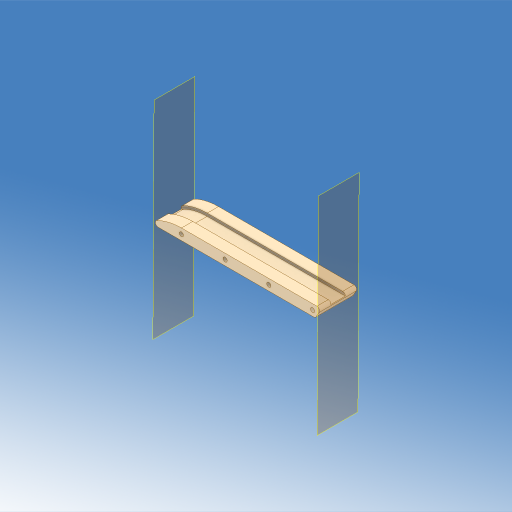
# Autodesk Inventor part: chain guide
Saved by Autodesk Inventor 2024 (Build 280153000, 153)
## iProperties
Created: 2023-03-01
Part Number: chain guide
Material: Polyethylene, High Density
Document SubType Name: Modeling
Designer: ralph
Density: 0.952 g/cm^3
Appearance: Smooth - Off-White
Author: ralph
Autodesk Inventor part; units mm, degrees
(part 1 of 2)
ref_plane "YZ Plane" through (0, 0, 0) normal (1, 0, 0) x (0, 1, 0)
ref_plane "XZ Plane" through (0, 0, 0) normal (0, 1, 0) x (-1, 0, 0)
ref_plane "XY Plane" through (0, 0, 0) normal (0, 0, 1) x (1, 0, 0)
ref_plane "Work Plane1" through (161.725, -21.8362, 0) normal (0, 0, 1) x (-0.4541702, 0.8909149, 0)
ref_plane "Work Plane2" through (-185.3421, -221.2521, 43.0784) normal (0, 0, -1) x (-0.1993348, 0.9799314, 0)
sketch "Sketch1" plane through (161.725, -21.8362, 0) normal (0, 0, 1) x (-0.4541702, 0.8909149, 0)
  circle A0 centre (-25.198, 87.6805) radius 3.175 projected
  line L0 (-137.9602, 56.9328) -> (35.8157, 235.3516) projected
  line L1 (82.5479, 91.7802) -> (42.7331, 68.5436) projected
  line L2 (134.3813, 156.1871) -> (107.8298, 115.7603) projected
  line L3 (-111.1407, 21.5887) -> (-101.5062, 29.8628) projected
  line L4 (-105.6433, 34.6801) -> (-115.2779, 26.406) projected
  line L5 (-3.5943, 192.0403) -> (-4.3034, 192.7309) projected
  line L6 (-3.5943, 192.0403) -> (-10.2226, 185.2349) projected
  line L7 (-10.9317, 185.9255) -> (-10.2226, 185.2349) projected
  arc A1 (2.942, 134.7748) -> (-78.867, 82.7393) centre (-35.4691, 104.837) ccw
  line L8 (2.942, 134.7748) -> (32.6751, 96.6265)
  arc A2 (44.4149, 71.1206) -> (32.6751, 96.6265) centre (-15.7529, 58.8814) ccw
  line L9 (44.4149, 71.1206) -> (83.6822, -121.9177)
  arc A3 (34.1459, -139.2082) -> (83.6822, -121.9177) centre (57.7385, -127.1951) ccw
  line L10 (34.1459, -139.2082) -> (-78.867, 82.7393)
  line L11 (86.7935, -121.2849) -> (47.5262, 71.7534)
  arc A4 (47.5262, 71.7534) -> (35.1793, 98.5783) centre (-15.7529, 58.8814) ccw
  line L12 (35.1793, 98.5783) -> (5.4462, 136.7266)
  arc A5 (5.4462, 136.7266) -> (-81.6964, 81.2986) centre (-35.4691, 104.837) ccw
  line L13 (-81.6964, 81.2986) -> (31.3166, -140.6489)
  arc A6 (31.3166, -140.6489) -> (86.7935, -121.2849) centre (57.7385, -127.1951) ccw
  line L14 (74.3484, -123.8164) -> (35.0811, 69.2219)
  arc A7 (35.0811, 69.2219) -> (25.1625, 90.7711) centre (-15.7529, 58.8814) ccw
  line L15 (25.1625, 90.7711) -> (-4.5706, 128.9194)
  arc A8 (-4.5706, 128.9194) -> (-70.379, 87.0612) centre (-35.4691, 104.837) ccw
  line L16 (-70.379, 87.0612) -> (42.6339, -134.8862)
  arc A9 (42.6339, -134.8862) -> (74.3484, -123.8164) centre (57.7385, -127.1951) ccw
  arc A10 (5.8406, 137.034) -> (-82.1419, 81.0717) centre (-35.4691, 104.837) ccw
  line L17 (5.8406, 137.034) -> (35.5737, 98.8857)
  arc A11 (48.0162, 71.8531) -> (35.5737, 98.8857) centre (-15.7529, 58.8814) ccw
  line L18 (48.0162, 71.8531) -> (87.2835, -121.1852)
  arc A12 (30.871, -140.8757) -> (87.2835, -121.1852) centre (57.7385, -127.1951) ccw
  line L19 (30.871, -140.8757) -> (-82.1419, 81.0717)
  line L20 (35.0811, 69.2219) -> (26.9658, 109.1164)
  circle A13 centre (57.7385, -127.1951) radius 44.45
  line L21 (76.5649, -86.9289) -> (65.8232, -81.9066)
  line L22 (5.092, 163.5049) -> (21.707, 97.431) projected
  line L23 (16.9598, 93.9553) -> (-30.1799, 123.0636) projected
  line L24 (-32.8692, 137.5188) -> (-4.5914, 166.5521) projected
  line L25 (29.8165, 96.4279) -> (15.4242, 153.6621) projected
  line L26 (20.7934, 156.6354) -> (60.85, 114.9227) projected
  line L27 (59.7201, 100.498) -> (42.2664, 90.3117) projected
  line L28 (16.7525, 188.4662) -> (29.5545, 201.6103) projected
  line L29 (102.7916, 142.7886) -> (91.8918, 126.1928) projected
  line L30 (66.3462, 120.2006) -> (40.7971, 146.806) projected
  line L31 (-106.6065, 61.8114) -> (-103.8347, 64.6572) projected
  line L32 (-88.1733, 62.7788) -> (-84.3051, 57.8167) projected
  line L33 (-71.9024, 23.6808) -> (-75.2673, 21.717) projected
  line L34 (-82.4286, 45.3973) -> (-80.2793, 47.2431) projected
  line L35 (-75.7066, 46.7865) -> (-69.9197, 39.3629) projected
  line L36 (41.0185, 151.4137) -> (46.0865, 155.7661) projected
  line L37 (41.1219, 161.5468) -> (35.4645, 156.6883) projected
  line L38 (31.1059, 156.8978) -> (17.9326, 170.6158) projected
  line L39 (-84.7406, 53.4561) -> (-87.3932, 51.1781) projected
  arc A14 (19.6429, 91.6626) -> (21.4459, 90.8569) centre (24.9298, 101.0743) ccw projected
  arc A15 (23.5785, 87.5163) -> (21.4459, 90.8569) centre (20.4213, 87.8518) ccw projected
  arc A16 (23.5785, 87.5163) -> (24.0318, 82.5663) centre (36.1917, 86.1757) ccw projected
  arc A17 (22.7005, 78.9892) -> (24.0318, 82.5663) centre (20.9881, 81.6628) ccw projected
  line L40 (22.7005, 78.9892) -> (6.0457, 68.3219) projected
  arc A18 (2.2151, 68.6304) -> (6.0457, 68.3219) centre (4.3333, 70.9955) ccw projected
  arc A19 (2.2151, 68.6304) -> (-6.0801, 71.8722) centre (-6.2676, 59.1587) ccw projected
  arc A20 (-8.9054, 73.6936) -> (-6.0801, 71.8722) centre (-6.0333, 75.0469) ccw projected
  line L41 (-8.9054, 73.6936) -> (-12.8049, 81.9696) projected
  arc A21 (-12.9858, 84.1944) -> (-12.8049, 81.9696) centre (-9.9328, 83.3229) ccw projected
  arc A22 (-12.9858, 84.1944) -> (-20.1115, 99.3174) centre (-25.198, 87.6805) ccw projected
  arc A23 (-21.712, 100.8733) -> (-20.1115, 99.3174) centre (-18.8398, 102.2266) ccw projected
  line L42 (-21.712, 100.8733) -> (-28.5783, 115.4459) projected
  arc A24 (-26.3647, 117.5067) -> (-28.5783, 115.4459) centre (-27.1422, 116.1226) ccw projected
  line L43 (-26.3647, 117.5067) -> (19.6429, 91.6626) projected
  line L44 (-65.6079, 77.0105) -> (-80.7722, 80.8743) projected
  line L45 (-82.4908, 86.5713) -> (-54.2131, 115.6046) projected
  line L46 (-42.2841, 112.6957) -> (-42.2475, 112.609) projected
  line L47 (-99.9792, 13.6685) -> (-98.0354, 10.338) projected
  line L48 (118.4433, 166.6195) -> (116.9435, 164.3359) projected
  line L49 (-124.3285, 43.6159) -> (-123.0701, 44.9079) projected
  line L50 (-120.8252, 44.9375) -> (-116.1944, 40.4272) projected
  line L51 (-43.1046, 108.967) -> (-65.0617, 90.1102) projected
  line L52 (-65.4017, 85.633) -> (-62.4154, 82.1557) projected
  ellipse E0 centre (81.3052, 191.0464) end of major axis (135.8081, 158.463) minor radius 63.4993 (134.3813, 156.1871) -> (35.8157, 235.3516) ccw projected
  ellipse E1 centre (44.1384, 157.5915) end of major axis (-21.2652, 196.6916) minor radius 76.1992 (82.5479, 91.7802) -> (107.8298, 115.7603) ccw projected
  ellipse E2 centre (-113.2093, 23.9973) end of major axis (-115.9344, 25.6265) minor radius 3.175 (-115.2779, 26.406) -> (-111.1407, 21.5887) ccw projected
  ellipse E3 centre (-103.5747, 32.2715) end of major axis (-106.2999, 33.9007) minor radius 3.175 (-101.5062, 29.8628) -> (-105.6433, 34.6801) ccw projected
  ellipse E4 centre (5.3104, 178.2592) end of major axis (-5.5902, 184.7759) minor radius 12.6999 (-0.7915, 167.1213) -> (2.6724, 165.8363) ccw projected
  ellipse E5 centre (2.0128, 162.7306) end of major axis (-0.7123, 164.3598) minor radius 3.175 (5.092, 163.5049) -> (2.6724, 165.8363) ccw projected
  ellipse E6 centre (18.6279, 96.6567) end of major axis (21.3531, 95.0276) minor radius 3.175 (16.9598, 93.9553) -> (21.707, 97.431) ccw projected
  ellipse E7 centre (-28.5118, 125.765) end of major axis (-25.7867, 124.1359) minor radius 3.175 (-31.6717, 126.0744) -> (-30.1799, 123.0636) ccw projected
  ellipse E8 centre (-44.3112, 127.3117) end of major axis (-55.2118, 133.8284) minor radius 12.6999 (-31.6717, 126.0744) -> (-33.338, 133.7052) ccw projected
  ellipse E9 centre (-30.5947, 135.3035) end of major axis (-27.8696, 133.6744) minor radius 3.175 (-32.8692, 137.5188) -> (-33.338, 133.7052) ccw projected
  ellipse E10 centre (-2.317, 164.3368) end of major axis (-5.0421, 165.966) minor radius 3.175 (-0.7915, 167.1213) -> (-4.5914, 166.5521) ccw projected
  ellipse E11 centre (32.8956, 97.2021) end of major axis (35.6207, 95.5729) minor radius 3.175 (29.8165, 96.4279) -> (32.2361, 94.0964) ccw projected
  ellipse E12 centre (18.5034, 154.4363) end of major axis (15.7782, 156.0655) minor radius 3.175 (20.7934, 156.6354) -> (15.4242, 153.6621) ccw projected
  ellipse E13 centre (58.56, 112.7236) end of major axis (55.8348, 114.3528) minor radius 3.175 (61.5424, 111.6347) -> (60.85, 114.9227) ccw projected
  ellipse E14 centre (73.4722, 107.2793) end of major axis (62.5716, 113.7959) minor radius 12.6999 (61.5424, 111.6347) -> (61.1902, 104.048) ccw projected
  ellipse E15 centre (58.1197, 103.2401) end of major axis (60.8449, 101.611) minor radius 3.175 (59.7201, 100.498) -> (61.1902, 104.048) ccw projected
  ellipse E16 centre (40.666, 93.0538) end of major axis (43.3911, 91.4247) minor radius 3.175 (38.4524, 90.7778) -> (42.2664, 90.3117) ccw projected
  ellipse E17 centre (20.2226, 172.8149) end of major axis (22.9478, 171.1857) minor radius 3.175 (17.2402, 173.9037) -> (17.9326, 170.6158) ccw projected
  ellipse E18 centre (5.3104, 178.2592) end of major axis (-5.5902, 184.7759) minor radius 12.6999 (17.2402, 173.9037) -> (16.2836, 184.6526) ccw projected
  ellipse E19 centre (19.0269, 186.251) end of major axis (21.7521, 184.6218) minor radius 3.175 (16.7525, 188.4662) -> (16.2836, 184.6526) ccw projected
  ellipse E20 centre (31.829, 199.395) end of major axis (29.1038, 201.0242) minor radius 3.175 (34.9594, 198.865) -> (29.5545, 201.6103) ccw projected
  ellipse E21 centre (81.29, 191.021) end of major axis (40.9578, 215.1327) minor radius 46.9895 (50.2522, 155.7412) -> (98.9449, 147.474) ccw projected
  ellipse E22 centre (100.1378, 144.5316) end of major axis (97.4127, 146.1608) minor radius 3.175 (102.7916, 142.7886) -> (98.9449, 147.474) ccw projected
  ellipse E23 centre (44.1233, 157.5662) end of major axis (-4.9294, 186.8912) minor radius 57.1494 (85.1993, 117.8311) -> (91.8918, 126.1928) ccw projected
  ellipse E24 centre (82.9173, 120.0386) end of major axis (85.6425, 118.4094) minor radius 3.175 (81.0283, 117.4867) -> (85.1993, 117.8311) ccw projected
  ellipse E25 centre (73.4722, 107.2793) end of major axis (62.5716, 113.7959) minor radius 12.6999 (81.0283, 117.4867) -> (69.6034, 119.3756) ccw projected
  ellipse E26 centre (68.6362, 122.3997) end of major axis (71.3614, 120.7705) minor radius 3.175 (66.3462, 120.2006) -> (69.6034, 119.3756) ccw projected
  ellipse E27 centre (-108.4072, 28.109) end of major axis (-132.9335, 42.7716) minor radius 28.5747 (-80.0217, 24.8241) -> (-83.1647, 41.5007) ccw projected
  ellipse E28 centre (-104.332, 59.5961) end of major axis (-101.6068, 57.967) minor radius 3.175 (-106.6065, 61.8114) -> (-104.7395, 56.4474) ccw projected
  ellipse E29 centre (-101.5603, 62.4419) end of major axis (-104.2854, 64.0711) minor radius 3.175 (-100.0348, 65.2264) -> (-103.8347, 64.6572) ccw projected
  ellipse E30 centre (-93.9329, 76.3643) end of major axis (-83.0323, 69.8476) minor radius 12.6999 (-100.0348, 65.2264) -> (-91.3284, 63.9343) ccw projected
  ellipse E31 centre (-90.6773, 60.8268) end of major axis (-93.4025, 62.456) minor radius 3.175 (-88.1733, 62.7788) -> (-91.3284, 63.9343) ccw projected
  ellipse E32 centre (-72.4237, 37.4109) end of major axis (-75.1489, 39.0401) minor radius 3.175 (-69.569, 36.0211) -> (-69.9197, 39.3629) ccw projected
  ellipse E33 centre (-58.1503, 30.4621) end of major axis (-69.0509, 36.9787) minor radius 12.6999 (-69.569, 36.0211) -> (-70.4323, 27.2308) ccw projected
  ellipse E34 centre (-73.5028, 26.4229) end of major axis (-70.7776, 24.7938) minor radius 3.175 (-71.9024, 23.6808) -> (-70.4323, 27.2308) ccw projected
  ellipse E35 centre (-76.8677, 24.4591) end of major axis (-74.1426, 22.8299) minor radius 3.175 (-80.0217, 24.8241) -> (-75.2673, 21.717) ccw projected
  ellipse E36 centre (-108.4072, 28.109) end of major axis (-132.9335, 42.7716) minor radius 28.5747 (-91.3563, 51.0389) -> (-104.7395, 56.4474) ccw projected
  ellipse E37 centre (81.29, 191.021) end of major axis (40.9578, 215.1327) minor radius 46.9895 (34.9594, 198.865) -> (41.7265, 165.6685) ccw projected
  ellipse E38 centre (-80.36, 42.9886) end of major axis (-83.0851, 44.6178) minor radius 3.175 (-82.4286, 45.3973) -> (-83.1647, 41.5007) ccw projected
  ellipse E39 centre (-78.2107, 44.8345) end of major axis (-80.9358, 46.4636) minor radius 3.175 (-75.7066, 46.7865) -> (-80.2793, 47.2431) ccw projected
  ellipse E40 centre (43.0871, 149.0051) end of major axis (45.8123, 147.3759) minor radius 3.175 (41.0185, 151.4137) -> (40.7971, 146.806) ccw projected
  ellipse E41 centre (48.155, 153.3574) end of major axis (45.4299, 154.9866) minor radius 3.175 (50.2522, 155.7412) -> (46.0865, 155.7661) ccw projected
  ellipse E42 centre (33.3959, 159.0969) end of major axis (36.1211, 157.4678) minor radius 3.175 (31.1059, 156.8978) -> (35.4645, 156.6883) ccw projected
  ellipse E43 centre (39.0533, 163.9555) end of major axis (36.3282, 165.5846) minor radius 3.175 (41.1219, 161.5468) -> (41.7265, 165.6685) ccw projected
  ellipse E44 centre (-86.8092, 55.8647) end of major axis (-89.5343, 57.4939) minor radius 3.175 (-84.7406, 53.4561) -> (-84.3051, 57.8167) ccw projected
  ellipse E45 centre (-89.4617, 53.5867) end of major axis (-86.7366, 51.9575) minor radius 3.175 (-91.3563, 51.0389) -> (-87.3932, 51.1781) ccw projected
  ellipse E46 centre (-79.9882, 83.951) end of major axis (-77.2631, 82.3218) minor radius 3.175 (-82.7772, 82.4337) -> (-80.7722, 80.8743) ccw projected
  ellipse E47 centre (-93.9329, 76.3643) end of major axis (-104.8335, 82.881) minor radius 12.6999 (-82.7772, 82.4337) -> (-82.9597, 82.7577) ccw projected
  ellipse E48 centre (-80.2164, 84.3561) end of major axis (-77.4912, 82.7269) minor radius 3.175 (-82.4908, 86.5713) -> (-82.9597, 82.7577) ccw projected
  ellipse E49 centre (-51.9386, 113.3893) end of major axis (-54.6638, 115.0185) minor radius 3.175 (-50.4131, 116.1738) -> (-54.2131, 115.6046) ccw projected
  ellipse E50 centre (-44.3112, 127.3117) end of major axis (-33.4106, 120.7951) minor radius 12.6999 (-50.4131, 116.1738) -> (-45.03, 114.6322) ccw projected
  ellipse E51 centre (-45.2097, 111.4623) end of major axis (-47.9349, 113.0915) minor radius 3.175 (-42.2841, 112.6957) -> (-45.03, 114.6322) ccw projected
  ellipse E52 centre (69.1742, 230.4776) end of major axis (66.4491, 232.1067) minor radius 3.175 (71.8221, 228.7255) -> (68.2422, 233.5127) ccw projected
  ellipse E53 centre (87.7091, 218.2134) end of major axis (71.3582, 227.9884) minor radius 19.0498 (71.8221, 228.7255) -> (69.7676, 224.6169) ccw projected
  ellipse E54 centre (66.7773, 225.6842) end of major axis (69.5025, 224.055) minor radius 3.175 (65.4394, 222.8049) -> (69.7676, 224.6169) ccw projected
  ellipse E55 centre (57.412, 205.529) end of major axis (41.0611, 215.3041) minor radius 19.0498 (65.4394, 222.8049) -> (61.0705, 224.2242) ccw projected
  ellipse E56 centre (61.6803, 227.3401) end of major axis (64.4054, 225.7109) minor radius 3.175 (60.1718, 230.1339) -> (61.0705, 224.2242) ccw projected
  ellipse E57 centre (81.29, 191.021) end of major axis (119.4421, 168.2127) minor radius 44.4495 (68.2422, 233.5127) -> (60.1718, 230.1339) ccw projected
  ellipse E58 centre (115.0715, 214.7362) end of major axis (117.7966, 213.107) minor radius 3.175 (114.2234, 211.6765) -> (117.6701, 216.5604) ccw projected
  ellipse E59 centre (109.1353, 193.3188) end of major axis (92.7844, 203.0938) minor radius 19.0498 (114.2234, 211.6765) -> (109.681, 212.3609) ccw projected
  ellipse E60 centre (109.772, 215.5345) end of major axis (112.4971, 213.9054) minor radius 3.175 (106.6201, 215.9172) -> (109.681, 212.3609) ccw projected
  ellipse E61 centre (87.7091, 218.2134) end of major axis (71.3582, 227.9884) minor radius 19.0498 (106.6201, 215.9172) -> (106.6199, 220.5109) ccw projected
  ellipse E62 centre (109.7718, 220.8938) end of major axis (107.0466, 222.5229) minor radius 3.175 (111.9627, 223.1917) -> (106.6199, 220.5109) ccw projected
  ellipse E63 centre (81.29, 191.021) end of major axis (119.4421, 168.2127) minor radius 44.4495 (117.6701, 216.5604) -> (111.9627, 223.1917) ccw projected
  ellipse E64 centre (-99.4065, 9.5378) end of major axis (-98.0439, 8.7232) minor radius 1.5875 (-98.7141, 8.1092) -> (-98.0354, 10.338) ccw projected
  ellipse E65 centre (-108.4072, 28.109) end of major axis (-127.4832, 39.5132) minor radius 22.2248 (-107.6415, 5.8974) -> (-98.7141, 8.1092) ccw projected
  ellipse E66 centre (-107.7509, 9.0705) end of major axis (-110.476, 10.6997) minor radius 3.175 (-108.8456, 12.0508) -> (-107.6415, 5.8974) ccw projected
  ellipse E67 centre (-113.2245, 23.972) end of major axis (-102.3239, 17.4553) minor radius 12.6999 (-108.8456, 12.0508) -> (-104.822, 14.4489) ccw projected
  ellipse E68 centre (-102.7214, 12.0682) end of major axis (-99.9962, 10.439) minor radius 3.175 (-99.9792, 13.6685) -> (-104.822, 14.4489) ccw projected
  ellipse E69 centre (114.2897, 166.0789) end of major axis (117.0148, 164.4497) minor radius 3.175 (111.1169, 165.9603) -> (116.9435, 164.3359) ccw projected
  ellipse E70 centre (92.0803, 165.2488) end of major axis (75.7294, 175.0238) minor radius 19.0498 (111.1169, 165.9603) -> (110.359, 170.6139) ccw projected
  ellipse E71 centre (113.4055, 171.5081) end of major axis (110.6804, 173.1372) minor radius 3.175 (112.7955, 174.6239) -> (110.359, 170.6139) ccw projected
  ellipse E72 centre (109.1353, 193.3188) end of major axis (92.7844, 203.0938) minor radius 19.0498 (112.7955, 174.6239) -> (117.1643, 176.0436) ccw projected
  ellipse E73 centre (118.5024, 173.1643) end of major axis (115.7773, 174.7935) minor radius 3.175 (121.3649, 171.7907) -> (117.1643, 176.0436) ccw projected
  ellipse E74 centre (81.29, 191.021) end of major axis (119.4421, 168.2127) minor radius 44.4495 (118.4433, 166.6195) -> (121.3649, 171.7907) ccw projected
  ellipse E75 centre (-121.9329, 43.8002) end of major axis (-123.2954, 44.6148) minor radius 1.5875 (-120.8252, 44.9375) -> (-123.0701, 44.9079) ccw projected
  ellipse E76 centre (-117.302, 39.29) end of major axis (-118.6646, 40.1046) minor radius 1.5875 (-116.3137, 38.0477) -> (-116.1944, 40.4272) ccw projected
  ellipse E77 centre (-108.4072, 28.109) end of major axis (-119.3078, 34.6257) minor radius 12.6999 (-116.3137, 38.0477) -> (-118.8274, 35.3692) ccw projected
  ellipse E78 centre (-113.2245, 23.972) end of major axis (-102.3239, 17.4553) minor radius 12.6999 (-118.8274, 35.3692) -> (-124.3475, 30.1012) ccw projected
  ellipse E79 centre (-127.1283, 31.6335) end of major axis (-129.8534, 33.2627) minor radius 3.175 (-130.2485, 32.2209) -> (-124.3475, 30.1012) ccw projected
  ellipse E80 centre (-108.4072, 28.109) end of major axis (-127.4832, 39.5132) minor radius 22.2248 (-124.3285, 43.6159) -> (-130.2485, 32.2209) ccw projected
  ellipse E81 centre (29.598, 81.6735) end of major axis (18.6974, 88.1902) minor radius 12.6999 (38.4524, 90.7778) -> (32.2361, 94.0964) ccw projected
  ellipse E82 centre (-62.9931, 87.7016) end of major axis (-60.2679, 86.0724) minor radius 3.175 (-65.0617, 90.1102) -> (-65.4017, 85.633) ccw projected
  ellipse E83 centre (-64.824, 80.0872) end of major axis (-62.0989, 78.458) minor radius 3.175 (-65.6079, 77.0105) -> (-62.4154, 82.1557) ccw projected
  ellipse E84 centre (-48.9751, 61.6327) end of major axis (-51.7002, 63.2618) minor radius 3.175 (-46.5664, 63.7012) -> (-48.1912, 64.7093) ccw projected
  line L53 (-46.5664, 63.7012) -> (-45.0469, 61.9319) projected
  ellipse E85 centre (-42.6383, 64.0005) end of major axis (-39.9132, 62.3713) minor radius 3.175 (-45.0469, 61.9319) -> (-40.6714, 61.5081) ccw projected
  ellipse E86 centre (-38.7045, 59.0157) end of major axis (-35.9794, 57.3866) minor radius 3.175 (-37.9206, 62.0924) -> (-40.6714, 61.5081) ccw projected
  line L54 (-37.9206, 62.0924) -> (-29.3488, 59.9083) projected
  line L55 (-78.8602, 72.5238) -> (-48.1912, 64.7093) projected
  ellipse E87 centre (2.465, 188.3722) end of major axis (0.5563, 189.5157) minor radius 2.225 projected
  ellipse E88 centre (-6.396, 179.2744) end of major axis (-4.4874, 178.1309) minor radius 2.225 projected
  ellipse E89 centre (-6.396, 179.2744) end of major axis (-11.4572, 182.3067) minor radius 5.8999 (-10.8256, 183.1717) -> (-0.6248, 178.0483) ccw projected
  ellipse E90 centre (5.2441, 176.8013) end of major axis (10.3911, 173.7176) minor radius 5.9999 (3.8429, 182.6354) -> (-0.6248, 178.0483) ccw projected
  ellipse E91 centre (2.465, 188.3722) end of major axis (-2.5962, 191.4045) minor radius 5.8999 (3.8429, 182.6354) -> (-1.5477, 192.6974) ccw projected
  ellipse E92 centre (-2.908, 194.1636) end of major axis (-4.6236, 195.1915) minor radius 2 (-4.3034, 192.7309) -> (-1.5477, 192.6974) ccw projected
  ellipse E93 centre (-12.3272, 184.4928) end of major axis (-10.6115, 183.4649) minor radius 2 (-10.8256, 183.1717) -> (-10.9317, 185.9255) ccw projected
  ellipse E94 centre (-108.392, 28.1344) end of major axis (-72.9651, 6.9552) minor radius 41.2746 (-137.9602, 56.9328) -> (-87.5869, -7.5134) ccw projected
  arc A25 (42.7331, 68.5436) -> (42.2932, 68.2869) centre (41.3036, 70.4877) ccw projected
  circle A26 centre (-43.1479, 88.299) radius 12.7 projected
  ellipse E95 centre (-45.1732, 111.3756) end of major axis (-47.8983, 113.0048) minor radius 3.175 (-43.1046, 108.967) -> (-42.2475, 112.609) ccw projected
  ellipse E96 centre (-30.1327, 56.8316) end of major axis (-32.8579, 58.4608) minor radius 3.175 (-26.9614, 56.6789) -> (-29.3488, 59.9083) ccw projected
  line L56 (42.2932, 68.2869) -> (-87.5869, -7.5134) projected
  ellipse E97 centre (-14.2761, 56.0678) end of major axis (-25.1767, 62.5845) minor radius 12.6999 (-26.9614, 56.6789) -> (-26.5581, 52.8365) ccw projected
  ellipse E98 centre (-29.6286, 52.0287) end of major axis (-26.9035, 50.3995) minor radius 3.175 (-28.0282, 49.2865) -> (-26.5581, 52.8365) ccw projected
  line L57 (-28.0282, 49.2865) -> (-45.482, 39.1002) projected
  ellipse E99 centre (-47.0824, 41.8423) end of major axis (-44.3572, 40.2132) minor radius 3.175 (-49.296, 39.5663) -> (-45.482, 39.1002) ccw projected
  ellipse E100 centre (-58.1503, 30.4621) end of major axis (-69.0509, 36.9787) minor radius 12.6999 (-49.296, 39.5663) -> (-60.7548, 42.8921) ccw projected
  ellipse E101 centre (-61.4059, 45.9996) end of major axis (-58.6808, 44.3704) minor radius 3.175 (-63.9099, 44.0476) -> (-60.7548, 42.8921) ccw projected
  line L58 (-63.9099, 44.0476) -> (-82.1636, 67.4635) projected
  ellipse E102 centre (-79.6595, 69.4155) end of major axis (-76.9344, 67.7863) minor radius 3.175 (-82.5142, 70.8052) -> (-82.1636, 67.4635) ccw projected
  ellipse E103 centre (-93.9329, 76.3643) end of major axis (-83.0323, 69.8476) minor radius 12.6999 (-82.5142, 70.8052) -> (-82.5019, 70.8306) ccw projected
  ellipse E104 centre (-79.6441, 69.4471) end of major axis (-76.919, 67.818) minor radius 3.175 (-78.8602, 72.5238) -> (-82.5019, 70.8306) ccw projected
  point P0 (92.9048, 134.1658)
  point P1 (66.1574, -83.5497)
  point P2 (80.1923, -88.8333)
  point P3 (-35.4703, 104.8623)
  point P4 (57.7373, -127.1698)
  dimension "d3" = 88.9
  dimension "d0" = 3.175
  dimension "d2" = 12.7
  constraints: 28 end point, 24 point on circle, 12 centre point, 3 point on line, 1 coincident, 1 collinear, 131 other
  measures "d0" distance between parallel lines of L9 L11
  measures "d2" distance between parallel lines of L11 L14
extrude "Extrusion1" add sketch "Sketch1" along normal up to surface (43.0784 mm away) contours A13 L9 L1 L11 | L56 A25 L1 L9 L21 L14 | L14 L20 L25 E11 E81 A2 L9 L1 A25 L56 | L14 L21 A13 | L1 L9 A2 E81 E16 A4 L11 | L20 L12 A4 E16 E81 A2 L8 | L8 A2 E81 E11 L25 L20
fillet "Fillet1" radius 3.175 1 edges at (52.2645, -47.3693, 21.5392)
ref_plane "Work Plane3" through (204.4469, 89.9538, 21.5392) normal (0, 0, 1) x (-0.622646, 0.7825036, 0)
sketch "Sketch3" plane through (204.4469, 89.9538, 21.5392) normal (0, 0, 1) x (-0.622646, 0.7825036, 0)
  line L0 (-184.7381, 186.3043) -> (21.1154, 326.503) projected
  line L1 (38.291, 176.4975) -> (-148.2221, 113.1103) projected
  line L2 (101.9227, 229.2796) -> (67.8456, 194.9568) projected
  line L3 (-168.5961, 151.8687) -> (-157.5055, 158.0564) projected
  line L4 (-154.4116, 152.5111) -> (-165.5022, 146.3234) projected
  line L5 (-121.6496, 199.8402) -> (-55.1465, -40.1805)
  arc A0 (-55.1465, -40.1805) -> (-3.1929, -33.1162) centre (-29.65, -33.1162) ccw
  line L6 (-3.1929, -33.1162) -> (-3.1929, 163.8755)
  arc A1 (-3.1929, 163.8755) -> (-9.611, 191.2017) centre (-64.575, 163.8755) ccw
  line L7 (-9.611, 191.2017) -> (-31.1431, 234.5113)
  arc A2 (-31.1431, 234.5113) -> (-121.6496, 199.8402) centre (-74.735, 212.8389) ccw
  line L8 (-125.1888, 198.8596) -> (-58.6857, -41.1611)
  arc A3 (-58.6857, -41.1611) -> (0.4796, -33.1162) centre (-29.65, -33.1162) ccw
  line L9 (0.4796, -33.1162) -> (0.4796, 163.8755)
  arc A4 (0.4796, 163.8755) -> (-6.3225, 192.8367) centre (-64.575, 163.8755) ccw
  line L10 (-6.3225, 192.8367) -> (-27.8546, 236.1463)
  arc A5 (-27.8546, 236.1463) -> (-125.1888, 198.8596) centre (-74.735, 212.8389) ccw
  line L11 (0, 0) -> (0, 163.8755) projected
  arc A6 (0, 0) -> (-12.7, 7.9752) centre (-29.65, -33.1162) ccw projected
  arc A7 (0, 163.8755) -> (-6.6784, 192.4746) centre (-64.575, 163.8755) ccw projected
  arc A8 (-6.6784, 192.4746) -> (-12.7, 191.0684) centre (-9.525, 191.0684) ccw projected
  line L12 (-12.7, 191.0684) -> (-12.7, 7.9752) projected
  line L13 (0, 0) -> (-3.1929, 2.2689)
  line L14 (-3.1929, 2.6025) -> (-3.1929, 163.8755)
  line L15 (-65.6726, 244.3466) -> (-32.1751, 267.1605) projected
  line L16 (-126.6144, 140.5738) -> (-130.3033, 139.3202) projected
  line L17 (-153.0212, 184.857) -> (-149.7379, 187.0931) projected
  line L18 (68.3161, 222.4688) -> (54.3269, 208.3787) projected
  line L19 (17.679, 189.6125) -> (-1.455, 183.1097) projected
  line L20 (-30.4188, 173.2663) -> (-49.5528, 166.7635) projected
  line L21 (-123.6965, 189.8236) -> (-95.2006, 176.0525) projected
  line L22 (-78.5166, 156.9201) -> (-97.6506, 150.4173) projected
  line L23 (-114.7225, 158.9387) -> (-127.9422, 185.5233) projected
  line L24 (-65.5928, 218.8876) -> (-28.5919, 184.15) projected
  line L25 (-62.7617, 175.5508) -> (-64.1496, 182.4577) projected
  line L26 (-69.3588, 208.3833) -> (-70.8787, 215.9475) projected
  line L27 (-79.8467, 221.8984) -> (-79.8282, 221.8061) projected
  line L28 (-109.8158, 191.5786) -> (-123.9055, 198.3877) projected
  line L29 (-124.4541, 204.3129) -> (-90.9565, 227.1268) projected
  line L30 (-134.7651, 182.1305) -> (-131.9637, 176.497) projected
  line L31 (28.0995, 207.5989) -> (8.3665, 238.7632) projected
  line L32 (-12.4358, 191.5849) -> (-15.1305, 250.5393) projected
  line L33 (-9.2763, 252.3828) -> (21.6616, 203.5225) projected
  line L34 (-23.2934, 262.2442) -> (-20.1826, 194.1844) projected
  line L35 (-25.5274, 191.7247) -> (-65.9188, 229.6454) projected
  line L36 (-133.2597, 172.3107) -> (-136.3131, 170.6071) projected
  line L37 (0.8815, 250.5843) -> (-9.293, 266.6528) projected
  line L38 (11.6232, 253.1434) -> (5.1109, 249.5101) projected
  line L39 (-132.6005, 163.9528) -> (-130.1263, 165.3331) projected
  line L40 (-125.7365, 163.9741) -> (-121.5455, 155.546) projected
  line L41 (9.502, 243.2343) -> (15.3358, 246.4891) projected
  line L42 (-174.0146, 170.5592) -> (-172.5239, 171.5744) projected
  line L43 (-170.3182, 171.156) -> (-166.6794, 165.8131) projected
  line L44 (-156.1236, 136.3592) -> (-154.8827, 132.708) projected
  line L45 (88.404, 242.7015) -> (86.4791, 240.7627) projected
  line L46 (-81.394, 218.4081) -> (-106.6692, 204.3065) projected
  line L47 (-107.8949, 199.987) -> (-105.6617, 195.9842) projected
  line L48 (-85.6578, 171.4408) -> (-77.6934, 167.5919) projected
  line L49 (-93.8094, 174.7408) -> (-92.6731, 172.7041) projected
  line L50 (-59.8451, 191.0194) -> (-69.0187, 207.4618) projected
  line L51 (-62.5837, 185.8558) -> (-61.0708, 186.6999) projected
  ellipse E0 centre (0.0819, 301.4333) end of major axis (-4.2511, 305.4378) minor radius 5.8999 (0.2886, 295.537) -> (-2.9881, 306.4717) ccw projected
  ellipse E1 centre (0.0779, 301.429) end of major axis (1.7119, 299.9189) minor radius 2.225 projected
  ellipse E2 centre (-161.5039, 152.1899) end of major axis (-131.0096, 124.3739) minor radius 41.2746 (-184.7381, 186.3043) -> (-148.2221, 113.1103) ccw projected
  ellipse E3 centre (13.7708, 248.6444) end of major axis (-42.5262, 299.997) minor radius 76.1992 (38.291, 176.4975) -> (67.8456, 194.9568) ccw projected
  ellipse E4 centre (56.8604, 274.0192) end of major axis (103.7746, 231.2254) minor radius 63.4993 (101.9227, 229.2796) -> (21.1154, 326.503) ccw projected
  ellipse E5 centre (-155.9586, 155.2837) end of major axis (-158.3043, 157.4234) minor radius 3.175 (-154.4116, 152.5111) -> (-157.5055, 158.0564) ccw projected
  ellipse E6 centre (-167.0491, 149.0961) end of major axis (-169.3948, 151.2358) minor radius 3.175 (-168.5961, 151.8687) -> (-165.5022, 146.3234) ccw projected
  ellipse E7 centre (-137.7011, 196.5915) end of major axis (-147.0839, 205.1503) minor radius 12.6999 (-145.9007, 186.8934) -> (-137.6266, 183.8918) ccw projected
  ellipse E8 centre (-111.7866, 144.4778) end of major axis (-102.4037, 135.919) minor radius 12.6999 (-101.2951, 151.6343) -> (-111.861, 157.1775) ccw projected
  ellipse E9 centre (-127.6361, 143.58) end of major axis (-125.2904, 141.4403) minor radius 3.175 (-126.6144, 140.5738) -> (-124.4662, 143.7595) ccw projected
  ellipse E10 centre (-131.3249, 142.3263) end of major axis (-128.9792, 140.1866) minor radius 3.175 (-134.3428, 143.3127) -> (-130.3033, 139.3202) ccw projected
  ellipse E11 centre (-151.234, 182.2328) end of major axis (-148.8883, 180.0931) minor radius 3.175 (-153.0212, 184.857) -> (-152.261, 179.2285) ccw projected
  ellipse E12 centre (-147.9506, 184.4689) end of major axis (-150.2963, 186.6086) minor radius 3.175 (-145.9007, 186.8934) -> (-149.7379, 187.0931) ccw projected
  ellipse E13 centre (-78.9197, 236.6252) end of major axis (-69.5369, 228.0664) minor radius 12.6999 (-66.7804, 232.8932) -> (-66.8923, 240.703) ccw projected
  ellipse E14 centre (-63.8854, 241.7224) end of major axis (-61.5397, 239.5827) minor radius 3.175 (-65.6726, 244.3466) -> (-66.8923, 240.703) ccw projected
  ellipse E15 centre (-30.3878, 264.5363) end of major axis (-32.7335, 266.676) minor radius 3.175 (-28.3379, 266.9608) -> (-32.1751, 267.1605) ccw projected
  ellipse E16 centre (-20.1383, 276.6589) end of major axis (-10.7554, 268.1001) minor radius 12.6999 (-28.3379, 266.9608) -> (-25.1997, 265.0112) ccw projected
  ellipse E17 centre (56.8604, 274.0192) end of major axis (91.5769, 242.3518) minor radius 46.9895 (19.413, 245.6343) -> (65.4806, 227.8269) ccw projected
  ellipse E18 centre (66.063, 224.7058) end of major axis (63.7173, 226.8455) minor radius 3.175 (68.3161, 222.4688) -> (65.4806, 227.8269) ccw projected
  ellipse E19 centre (13.7708, 248.6444) end of major axis (-28.4519, 287.1588) minor radius 57.1494 (46.1019, 201.5188) -> (54.3269, 208.3787) ccw projected
  ellipse E20 centre (44.3058, 204.1369) end of major axis (46.6515, 201.9972) minor radius 3.175 (41.946, 202.0128) -> (46.1019, 201.5188) ccw projected
  ellipse E21 centre (32.5068, 193.5164) end of major axis (41.8897, 184.9576) minor radius 12.6999 (21.6847, 200.1625) -> (19.8272, 192.7982) ccw projected
  ellipse E22 centre (16.6573, 192.6186) end of major axis (19.003, 190.4789) minor radius 3.175 (17.679, 189.6125) -> (19.8272, 192.7982) ccw projected
  ellipse E23 centre (-2.4766, 186.1159) end of major axis (-0.1309, 183.9762) minor radius 3.175 (-5.0995, 184.3267) -> (-1.455, 183.1097) ccw projected
  ellipse E24 centre (-15.591, 177.1702) end of major axis (-6.2081, 168.6114) minor radius 12.6999 (-5.0995, 184.3267) -> (-10.5295, 188.8179) ccw projected
  ellipse E25 centre (-31.4405, 176.2724) end of major axis (-29.0948, 174.1327) minor radius 3.175 (-30.4188, 173.2663) -> (-28.2706, 176.452) ccw projected
  ellipse E26 centre (-50.5744, 169.7696) end of major axis (-48.2287, 167.63) minor radius 3.175 (-53.1973, 167.9805) -> (-49.5528, 166.7635) ccw projected
  ellipse E27 centre (-79.0749, 164.7332) end of major axis (-81.4206, 166.8729) minor radius 3.175 (-75.9976, 163.9514) -> (-77.6934, 167.5919) ccw projected
  ellipse E28 centre (-63.6888, 160.824) end of major axis (-54.3059, 152.2652) minor radius 12.6999 (-75.9976, 163.9514) -> (-76.3684, 160.1057) ccw projected
  ellipse E29 centre (-79.5383, 159.9262) end of major axis (-77.1926, 157.7865) minor radius 3.175 (-78.5166, 156.9201) -> (-76.3684, 160.1057) ccw projected
  ellipse E30 centre (-98.6722, 153.4234) end of major axis (-96.3265, 151.2837) minor radius 3.175 (-101.2951, 151.6343) -> (-97.6506, 150.4173) ccw projected
  ellipse E31 centre (-111.8796, 160.3524) end of major axis (-109.5339, 158.2127) minor radius 3.175 (-114.7225, 158.9387) -> (-111.861, 157.1775) ccw projected
  ellipse E32 centre (-63.6888, 160.824) end of major axis (-54.3059, 152.2652) minor radius 12.6999 (-53.1973, 167.9805) -> (-60.4569, 173.1058) ccw projected
  ellipse E33 centre (-59.649, 176.1762) end of major axis (-57.3033, 174.0365) minor radius 3.175 (-62.7617, 175.5508) -> (-60.4569, 173.1058) ccw projected
  ellipse E34 centre (-67.766, 216.5729) end of major axis (-70.1117, 218.7126) minor radius 3.175 (-65.5928, 218.8876) -> (-70.8787, 215.9475) ccw projected
  ellipse E35 centre (-122.524, 201.2463) end of major axis (-120.1783, 199.1066) minor radius 3.175 (-125.5594, 200.3154) -> (-123.9055, 198.3877) ccw projected
  ellipse E36 centre (-137.7011, 196.5915) end of major axis (-128.3183, 188.0328) minor radius 12.6999 (-125.5594, 200.3154) -> (-125.6737, 200.6693) ccw projected
  ellipse E37 centre (-122.6668, 201.6887) end of major axis (-120.3211, 199.549) minor radius 3.175 (-124.4541, 204.3129) -> (-125.6737, 200.6693) ccw projected
  ellipse E38 centre (-89.1692, 224.5026) end of major axis (-91.5149, 226.6423) minor radius 3.175 (-87.1193, 226.9271) -> (-90.9565, 227.1268) ccw projected
  ellipse E39 centre (-78.9197, 236.6252) end of major axis (-88.3025, 245.184) minor radius 12.6999 (-87.1193, 226.9271) -> (-82.1515, 224.3434) ccw projected
  ellipse E40 centre (-82.9595, 221.273) end of major axis (-85.3052, 223.4127) minor radius 3.175 (-79.8467, 221.8984) -> (-82.1515, 224.3434) ccw projected
  ellipse E41 centre (-111.7866, 144.4778) end of major axis (-102.4037, 135.919) minor radius 12.6999 (-121.868, 152.2014) -> (-124.4662, 143.7595) ccw projected
  ellipse E42 centre (-137.608, 180.7169) end of major axis (-139.9537, 182.8566) minor radius 3.175 (-134.7651, 182.1305) -> (-137.6266, 183.8918) ccw projected
  ellipse E43 centre (-124.3883, 154.1323) end of major axis (-126.7341, 156.272) minor radius 3.175 (-121.868, 152.2014) -> (-121.5455, 155.546) ccw projected
  ellipse E44 centre (-6.6105, 268.3513) end of major axis (-4.2648, 266.2116) minor radius 3.175 (-9.3161, 270.0128) -> (-9.293, 266.6528) ccw projected
  ellipse E45 centre (30.7819, 209.2973) end of major axis (33.1276, 207.1577) minor radius 3.175 (28.0995, 207.5989) -> (31.1269, 206.1412) ccw projected
  ellipse E46 centre (-9.2642, 191.7298) end of major axis (-6.9185, 189.5901) minor radius 3.175 (-12.4358, 191.5849) -> (-10.5295, 188.8179) ccw projected
  ellipse E47 centre (-11.9588, 250.6843) end of major axis (-14.3045, 252.824) minor radius 3.175 (-9.2763, 252.3828) -> (-15.1305, 250.5393) ccw projected
  ellipse E48 centre (18.9791, 201.824) end of major axis (16.6334, 203.9637) minor radius 3.175 (21.6847, 200.1625) -> (21.6616, 203.5225) ccw projected
  ellipse E49 centre (-26.4651, 262.0993) end of major axis (-28.8108, 264.239) minor radius 3.175 (-23.2934, 262.2442) -> (-25.1997, 265.0112) ccw projected
  ellipse E50 centre (-23.3543, 194.0394) end of major axis (-21.0085, 191.8998) minor radius 3.175 (-25.5274, 191.7247) -> (-20.1826, 194.1844) ccw projected
  ellipse E51 centre (-63.7456, 231.9601) end of major axis (-61.3999, 229.8205) minor radius 3.175 (-66.7804, 232.8932) -> (-65.9188, 229.6454) ccw projected
  ellipse E52 centre (-161.5039, 152.1899) end of major axis (-140.3925, 132.9327) minor radius 28.5747 (-134.3428, 143.3127) -> (-134.0986, 160.2811) ccw projected
  ellipse E53 centre (-161.5039, 152.1899) end of major axis (-140.3925, 132.9327) minor radius 28.5747 (-140.2244, 171.2608) -> (-152.261, 179.2285) ccw projected
  ellipse E54 centre (56.8604, 274.0192) end of major axis (91.5769, 242.3518) minor radius 46.9895 (13.0232, 290.9411) -> (13.0373, 257.0618) ccw projected
  ellipse E55 centre (-134.8066, 175.0833) end of major axis (-137.1523, 177.223) minor radius 3.175 (-133.2597, 172.3107) -> (-131.9637, 176.497) ccw projected
  ellipse E56 centre (-137.86, 173.3798) end of major axis (-135.5143, 171.2401) minor radius 3.175 (-140.2244, 171.2608) -> (-136.3131, 170.6071) ccw projected
  ellipse E57 centre (10.0762, 255.9161) end of major axis (7.7305, 258.0558) minor radius 3.175 (11.6232, 253.1434) -> (13.0373, 257.0618) ccw projected
  ellipse E58 centre (3.5639, 252.2827) end of major axis (5.9096, 250.1431) minor radius 3.175 (0.8815, 250.5843) -> (5.1109, 249.5101) ccw projected
  ellipse E59 centre (-30.765, 181.8352) end of major axis (-33.1107, 183.9749) minor radius 3.175 (-27.7302, 180.9022) -> (-28.5919, 184.15) ccw projected
  ellipse E60 centre (-128.5794, 162.5605) end of major axis (-130.9251, 164.7002) minor radius 3.175 (-125.7365, 163.9741) -> (-130.1263, 165.3331) ccw projected
  ellipse E61 centre (-131.0535, 161.1801) end of major axis (-133.3992, 163.3198) minor radius 3.175 (-132.6005, 163.9528) -> (-134.0986, 160.2811) ccw projected
  ellipse E62 centre (16.8827, 243.7164) end of major axis (14.537, 245.8561) minor radius 3.175 (19.413, 245.6343) -> (15.3358, 246.4891) ccw projected
  ellipse E63 centre (11.049, 240.4616) end of major axis (13.3947, 238.3219) minor radius 3.175 (9.502, 243.2343) -> (8.3665, 238.7632) ccw projected
  ellipse E64 centre (-161.5039, 152.1899) end of major axis (-177.9238, 167.1677) minor radius 22.2248 (-174.0146, 170.5592) -> (-182.0872, 160.573) ccw projected
  ellipse E65 centre (-171.6303, 170.2624) end of major axis (-172.8032, 171.3322) minor radius 1.5875 (-170.3182, 171.156) -> (-172.5239, 171.5744) ccw projected
  ellipse E66 centre (-167.9915, 164.9195) end of major axis (-169.1643, 165.9894) minor radius 1.5875 (-167.2706, 163.5051) -> (-166.6794, 165.8131) ccw projected
  ellipse E67 centre (-161.5039, 152.1899) end of major axis (-152.121, 143.6311) minor radius 12.6999 (-167.2706, 163.5051) -> (-170.2677, 161.3814) ccw projected
  ellipse E68 centre (-167.0491, 149.0961) end of major axis (-176.432, 157.6549) minor radius 12.6999 (-170.2677, 161.3814) -> (-176.7272, 157.3196) ccw projected
  ellipse E69 centre (-179.1467, 159.3754) end of major axis (-181.4924, 161.5151) minor radius 3.175 (-182.0872, 160.573) -> (-176.7272, 157.3196) ccw projected
  ellipse E70 centre (-159.1297, 135.3376) end of major axis (-156.784, 133.1979) minor radius 3.175 (-156.1236, 136.3592) -> (-160.7136, 138.0893) ccw projected
  ellipse E71 centre (-156.3857, 132.1972) end of major axis (-155.2129, 131.1274) minor radius 1.5875 (-155.992, 130.6593) -> (-154.8827, 132.708) ccw projected
  ellipse E72 centre (-161.5039, 152.1899) end of major axis (-177.9238, 167.1677) minor radius 22.2248 (-165.1811, 130.2714) -> (-155.992, 130.6593) ccw projected
  ellipse E73 centre (-164.6558, 133.4026) end of major axis (-167.0015, 135.5423) minor radius 3.175 (-165.1345, 136.5413) -> (-165.1811, 130.2714) ccw projected
  ellipse E74 centre (-167.0491, 149.0961) end of major axis (-176.432, 157.6549) minor radius 12.6999 (-165.1345, 136.5413) -> (-160.7136, 138.0893) ccw projected
  ellipse E75 centre (68.571, 299.3863) end of major axis (82.6453, 286.5482) minor radius 19.0498 (55.0983, 312.8544) -> (52.2661, 309.2377) ccw projected
  ellipse E76 centre (49.5486, 310.8796) end of major axis (51.8943, 308.7399) minor radius 3.175 (47.6635, 308.3248) -> (52.2661, 309.2377) ccw projected
  ellipse E77 centre (36.3535, 292.9958) end of major axis (50.4278, 280.1577) minor radius 19.0498 (47.6635, 308.3248) -> (43.6653, 310.5865) ccw projected
  ellipse E78 centre (44.8839, 313.5183) end of major axis (47.2296, 311.3786) minor radius 3.175 (43.9626, 316.5567) -> (43.6653, 310.5865) ccw projected
  ellipse E79 centre (56.8604, 274.0192) end of major axis (89.7003, 244.0636) minor radius 44.4495 (52.5445, 318.259) -> (43.9626, 316.5567) ccw projected
  ellipse E80 centre (52.8528, 315.099) end of major axis (50.5071, 317.2387) minor radius 3.175 (55.0983, 312.8544) -> (52.5445, 318.259) ccw projected
  ellipse E81 centre (84.6049, 270.7204) end of major axis (98.6791, 257.8822) minor radius 19.0498 (93.2503, 287.6954) -> (88.9354, 289.2715) ccw projected
  ellipse E82 centre (89.6572, 292.3633) end of major axis (92.0029, 290.2236) minor radius 3.175 (86.6449, 293.3666) -> (88.9354, 289.2715) ccw projected
  ellipse E83 centre (68.571, 299.3863) end of major axis (82.6453, 286.5482) minor radius 19.0498 (86.6449, 293.3666) -> (87.5604, 297.8681) ccw projected
  ellipse E84 centre (90.7252, 297.6151) end of major axis (88.3795, 299.7548) minor radius 3.175 (93.3302, 299.4301) -> (87.5604, 297.8681) ccw projected
  ellipse E85 centre (56.8604, 274.0192) end of major axis (89.7003, 244.0636) minor radius 44.4495 (97.6012, 291.7943) -> (93.3302, 299.4301) ccw projected
  ellipse E86 centre (94.6912, 290.5246) end of major axis (97.0369, 288.3849) minor radius 3.175 (93.2503, 287.6954) -> (97.6012, 291.7943) ccw projected
  ellipse E87 centre (56.8604, 274.0192) end of major axis (89.7003, 244.0636) minor radius 44.4495 (88.404, 242.7015) -> (92.2978, 247.1865) ccw projected
  ellipse E88 centre (84.226, 242.9997) end of major axis (86.5717, 240.86) minor radius 3.175 (81.0932, 243.5159) -> (86.4791, 240.7627) ccw projected
  ellipse E89 centre (62.2968, 246.6133) end of major axis (76.3711, 233.7752) minor radius 19.0498 (81.0932, 243.5159) -> (81.2782, 248.2272) ccw projected
  ellipse E90 centre (84.4418, 248.4961) end of major axis (82.0961, 250.6358) minor radius 3.175 (84.4651, 251.671) -> (81.2782, 248.2272) ccw projected
  ellipse E91 centre (84.6049, 270.7204) end of major axis (98.6791, 257.8822) minor radius 19.0498 (84.4651, 251.671) -> (89.0292, 252.1913) ccw projected
  ellipse E92 centre (89.7666, 249.1032) end of major axis (87.4208, 251.2429) minor radius 3.175 (92.2978, 247.1865) -> (89.0292, 252.1913) ccw projected
  ellipse E93 centre (-86.3214, 186.8641) end of major axis (-85.3831, 186.0082) minor radius 1.27 projected
  ellipse E94 centre (-75.2309, 193.0517) end of major axis (-74.2926, 192.1958) minor radius 1.27 projected
  ellipse E95 centre (-92.5092, 197.9547) end of major axis (-91.5709, 197.0988) minor radius 1.27 projected
  ellipse E96 centre (-81.4186, 204.1423) end of major axis (-80.4803, 203.2864) minor radius 1.27 projected
  ellipse E97 centre (-105.1223, 201.5339) end of major axis (-107.468, 203.6736) minor radius 3.175 (-106.6692, 204.3065) -> (-107.8949, 199.987) ccw projected
  ellipse E98 centre (-108.4343, 194.4373) end of major axis (-106.0886, 192.2976) minor radius 3.175 (-109.8158, 191.5786) -> (-105.6617, 195.9842) ccw projected
  ellipse E99 centre (-82.9409, 221.1807) end of major axis (-85.2867, 223.3204) minor radius 3.175 (-81.394, 218.4081) -> (-79.8282, 221.8061) ccw projected
  ellipse E100 centre (-96.5821, 173.1939) end of major axis (-98.9278, 175.3335) minor radius 3.175 (-93.8094, 174.7408) -> (-95.2006, 176.0525) ccw projected
  ellipse E101 centre (-89.9005, 174.251) end of major axis (-92.2462, 176.3907) minor radius 3.175 (-92.6731, 172.7041) -> (-88.4699, 171.4166) ccw projected
  ellipse E102 centre (-87.0392, 168.5822) end of major axis (-84.6935, 166.4425) minor radius 3.175 (-85.6578, 171.4408) -> (-88.4699, 171.4166) ccw projected
  ellipse E103 centre (32.5068, 193.5164) end of major axis (41.8897, 184.9576) minor radius 12.6999 (41.946, 202.0128) -> (31.1269, 206.1412) ccw projected
  ellipse E104 centre (-62.6177, 189.4725) end of major axis (-60.272, 187.3328) minor radius 3.175 (-61.0708, 186.6999) -> (-59.8451, 191.0194) ccw projected
  ellipse E105 centre (-66.2461, 209.0087) end of major axis (-63.9004, 206.869) minor radius 3.175 (-69.3588, 208.3833) -> (-69.0187, 207.4618) ccw projected
  ellipse E106 centre (-15.591, 177.1702) end of major axis (-6.2081, 168.6114) minor radius 12.6999 (-27.7302, 180.9022) -> (-28.2706, 176.452) ccw projected
  ellipse E107 centre (-61.0368, 183.0831) end of major axis (-63.3825, 185.2228) minor radius 3.175 (-62.5837, 185.8558) -> (-64.1496, 182.4577) ccw projected
  ellipse E108 centre (-20.1383, 276.6589) end of major axis (-10.7554, 268.1001) minor radius 12.6999 (-9.3161, 270.0128) -> (-8.1108, 280.7367) ccw projected
  ellipse E109 centre (-15.591, 177.1702) end of major axis (-14.6527, 176.3143) minor radius 1.27 projected
  ellipse E110 centre (-63.6888, 160.824) end of major axis (-62.7505, 159.9681) minor radius 1.27 projected
  ellipse E111 centre (32.5068, 193.5164) end of major axis (33.4451, 192.6605) minor radius 1.27 projected
  ellipse E112 centre (-111.7866, 144.4778) end of major axis (-110.8483, 143.6219) minor radius 1.27 projected
  ellipse E113 centre (-20.1383, 276.6589) end of major axis (-21.0766, 277.5148) minor radius 1.27 projected
  ellipse E114 centre (84.6049, 270.7204) end of major axis (83.6666, 271.5763) minor radius 1.27 projected
  ellipse E115 centre (68.571, 299.3863) end of major axis (67.6327, 300.2422) minor radius 1.27 projected
  ellipse E116 centre (-78.9197, 236.6252) end of major axis (-79.858, 237.4811) minor radius 1.27 projected
  ellipse E117 centre (32.4758, 260.3803) end of major axis (31.5375, 261.2362) minor radius 1.27 projected
  ellipse E118 centre (62.2968, 246.6133) end of major axis (61.3585, 247.4692) minor radius 1.27 projected
  ellipse E119 centre (36.3535, 292.9958) end of major axis (35.4152, 293.8517) minor radius 1.27 projected
  ellipse E120 centre (-137.7011, 196.5915) end of major axis (-138.6394, 197.4474) minor radius 1.27 projected
  ellipse E121 centre (56.8604, 274.0192) end of major axis (46.5393, 283.4339) minor radius 13.9698 projected
  ellipse E122 centre (-5.104, 281.7561) end of major axis (-2.7583, 279.6164) minor radius 3.175 (-6.8912, 284.3803) -> (-8.1108, 280.7367) ccw projected
  ellipse E123 centre (10.0612, 292.0845) end of major axis (7.7155, 294.2242) minor radius 3.175 (13.0232, 290.9411) -> (8.2739, 294.7087) ccw projected
  ellipse E124 centre (-125.0993, 186.937) end of major axis (-122.7536, 184.7973) minor radius 3.175 (-127.6197, 188.8679) -> (-127.9422, 185.5233) ccw projected
  ellipse E125 centre (-125.0779, 186.9649) end of major axis (-122.7322, 184.8252) minor radius 3.175 (-123.6965, 189.8236) -> (-127.6026, 188.8902) ccw projected
  ellipse E126 centre (-137.7011, 196.5915) end of major axis (-147.0839, 205.1503) minor radius 12.6999 (-127.6197, 188.8679) -> (-127.6026, 188.8902) ccw projected
  line L52 (-6.8912, 284.3803) -> (8.2739, 294.7087) projected
  point P0 (56.9089, 215.9898)
  point P1 (-10.9543, 193.9035)
  point P2 (-76.3213, 52.0927)
  point P3 (-102.0109, 140.7845)
  point P4 (-6.35, 163.8755)
  point P5 (-6.35, 113.0755)
  point P6 (-74.735, 212.8389)
  point P7 (-74.735, 212.8389)
  point P8 (-6.35, 113.0755)
  point P9 (-29.65, -33.1162)
  point P10 (-29.65, -33.1162)
  point P11 (-74.735, 212.8389)
  point P12 (-50.8349, 12.5336)
  point P13 (-50.8545, 12.5629)
  point P14 (-50.8349, 12.5336)
  point P15 (-50.8545, 12.5629)
  point P16 (-50.8349, 12.5336)
  point P17 (-50.8545, 12.5629)
  point P18 (-101.9993, 156.6594)
  point P19 (-106.8985, 174.3417)
  point P20 (-50.8349, 12.5336)
  point P21 (-50.8545, 12.5629)
  point P22 (-101.9993, 156.6594)
  point P23 (-106.8985, 174.3417)
  point P24 (-50.8349, 12.5336)
  point P25 (-50.8545, 12.5629)
  point P26 (-101.9993, 156.6594)
  point P27 (-106.8985, 174.3417)
  point P28 (-50.8349, 12.5336)
  point P29 (-50.8545, 12.5629)
  point P30 (-101.9993, 156.6594)
  point P31 (-106.8985, 174.3417)
  point P32 (-50.8349, 12.5336)
  point P33 (-50.8545, 12.5629)
  constraints: 16 end point, 13 point on circle, 6 centre point, 2 point on line, 131 other
extrude "Extrusion2" cut sketch "Sketch3" along normal blind 8.382 contours L6 A1 E24 E23 A7 L11 L1 | L1 L11 A6 L6 | A1 L7 A8 A7 E23 E24
sketch "Sketch4" plane through (204.4469, 89.9538, 21.5392) normal (0, 0, 1) x (-0.622646, 0.7825036, 0)
  line L0 (-3.1929, 163.8755) -> (-3.1929, 2.6025) projected
  arc A0 (-3.1929, 163.8755) -> (-9.611, 191.2017) centre (-64.575, 163.8755) ccw projected
  line L1 (-10.9543, 193.9035) -> (-9.611, 191.2017) projected
  arc A1 (-6.6784, 192.4746) -> (-10.9543, 193.9035) centre (-9.525, 191.0684) ccw projected
  arc A2 (0, 163.8755) -> (-6.6784, 192.4746) centre (-64.575, 163.8755) ccw projected
  line L2 (0, 0) -> (0, 163.8755) projected
  arc A3 (0, 0) -> (-3.1929, 2.6025) centre (-29.65, -33.1162) ccw projected
  point P0 (56.9089, 215.9898)
extrude "Extrusion3" cut sketch "Sketch4" against normal blind 8.382
sketch "Sketch5" plane through (204.4469, 89.9538, 43.0784) normal (0, 0, 1) x (-0.622646, 0.7825036, 0)
  arc A0 (-6.6784, 192.4746) -> (-12.7, 191.0684) centre (-9.525, 191.0684) ccw projected
  line L0 (-12.7, 191.0684) -> (-12.7, 7.9752) projected
  arc A1 (0, 0) -> (-12.7, 7.9752) centre (-29.65, -33.1162) ccw projected
  line L1 (0, 0) -> (0, 163.8755) projected
  arc A2 (0, 163.8755) -> (-6.6784, 192.4746) centre (-64.575, 163.8755) ccw projected
  arc A3 (0, 0) -> (-12.7, 7.9752) centre (-29.65, -33.1162) ccw projected
  line L2 (-12.7, 7.9752) -> (0, 7.9752) construction
  line L3 (0, 0) -> (0, 163.8755) projected
  line L4 (-6.35, 7.9752) -> (-6.35, 163.8755)
  circle A4 centre (-6.35, 163.8755) radius 2.413
  circle A5 centre (-6.35, 113.0755) radius 2.413
  circle A6 centre (-6.35, 62.2755) radius 2.413
  circle A7 centre (-6.35, 11.4755) radius 2.413
  point P0 (56.9089, 215.9898)
  dimension "d11" = 4.826
  dimension "d14" = 50.8
  constraints: 4 centre point, 4 coincident, 4 end point, 2 vertical, 1 midpoint, 1 perpendicular, 1 point on line, 9 other
  measures "d11" diameter of A4
  measures "d14" distance of A4.centre A5.centre
ref_plane "Work Plane4" through (-228.5882, -244.5835, 0) normal (0, 0, 1) x (1, 0, 0)
extrude "Extrusion4" cut sketch "Sketch5" against normal up to surface (43.0784 mm away) contours A7 L4 | L4 A7 | A6 L4 | L4 A6 | A5 L4 | L4 A5 | A4
thread "Thread1" size "10-24 UNC" class "2B" standard "ANSI Unified Screw Threads" full length
thread "Thread2" size "10-24 UNC" class "2B" standard "ANSI Unified Screw Threads" full length
thread "Thread3" size "10-24 UNC" class "2B" standard "ANSI Unified Screw Threads" full length
thread "Thread4" size "10-24 UNC" class "2B" standard "ANSI Unified Screw Threads" full length
fillet "Fillet2" radius 3.175 2 edges at (204.4469, 89.9538, 36.4998) (206.1139, 75.0502, 21.5392)
sketch "Sketch6" plane through (76.2138, -12.0827, 43.0784) normal (-0.622646, 0.7825036, 0) x (0, 0, -1)
  line L0 (29.9212, 30.0281) -> (29.9212, 28.5991) projected
  line L1 (29.9212, 28.5991) -> (43.0784, 28.5991) projected
  line L2 (43.0784, 28.5991) -> (43.0784, 27.193) projected
  line L3 (43.0784, 27.193) -> (0, 27.193) projected
  line L4 (0, 27.193) -> (0, 28.5991) projected
  line L5 (0, 28.5991) -> (13.1572, 28.5991) projected
  line L6 (13.1572, 28.5991) -> (13.1572, 30.0281) projected
  line L7 (13.1572, 30.0281) -> (29.9212, 30.0281) projected
  line L8 (0, -157.4036) -> (0, -160.0428) projected
  line L9 (0, -160.0428) -> (43.0784, -160.0428) projected
  line L10 (43.0784, -160.0428) -> (43.0784, -157.4036) projected
  line L11 (43.0784, -157.4036) -> (29.9212, -157.4036) projected
  line L12 (29.9212, -157.4036) -> (29.9212, -160.5785) projected
  line L13 (29.9212, -160.5785) -> (13.1572, -160.5785) projected
  line L14 (13.1572, -160.5785) -> (13.1572, -157.4036) projected
  line L15 (13.1572, -157.4036) -> (0, -157.4036) projected
  line L16 (0, 27.193) -> (0, 30.368) projected
  line L17 (43.0784, -160.5786) -> (0, -160.5786)
  line L18 (0, -160.5786) -> (0, 30.368)
  line L19 (0, 30.368) -> (43.0784, 30.368)
  line L20 (43.0784, 30.368) -> (43.0784, -160.5786)
  point P0 (43.0784, 52.1143)
  constraints: 8 end point, 2 parallel, 1 horizontal, 1 perpendicular
ref_plane "Work Plane5" through (203.8551, 85.4024, 0) normal (0.7860048, 0.6182204, 0) x (-0.6182204, 0.7860048, 0)